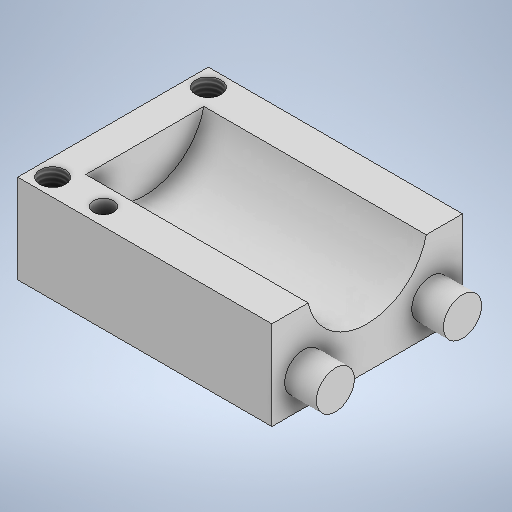
# Autodesk Inventor part: Rb oven housing bottom-back threaded
Saved by Autodesk Inventor 2025.3 (Build 293356000, 356)
## iProperties
Created: 2025-04-11
Part Number: Rb oven housing bottom-back threaded
Material: Generic
Document SubType Name: Modeling
Designer: Verðandi
Density: 1 g/cm^3
Appearance: Default
Author: Verðandi
Autodesk Inventor part; units mm, degrees
ref_plane "YZ Plane" through (0, 0, 0) normal (1, 0, 0) x (0, 1, 0)
ref_plane "XZ Plane" through (0, 0, 0) normal (0, 1, 0) x (-1, 0, 0)
ref_plane "XY Plane" through (0, 0, 0) normal (0, 0, 1) x (1, 0, 0)
sketch "Sketch1" plane through (0, 0, 0) normal (0, 0, 1) x (1, 0, 0)
  line L0 (20, -7) -> (-20, -7)
  line L1 (-20, -7) -> (-20, 7)
  line L2 (-20, 7) -> (20, 7)
  line L3 (20, 7) -> (20, -7)
  line L4 (20, -7) -> (-20, 7) construction
  line L5 (-20, -7) -> (20, 7) construction
  point P0 (0, 0)
  dimension "d0" = 40
  dimension "d1" = 14
  constraints: 12 end point, 2 midpoint, 2 parallel, 1 horizontal, 1 perpendicular
  measures "d0" distance of L1.end L2.end
  measures "d1" distance of L0.end L1.end
extrude "Extrusion1" add sketch "Sketch1" along normal blind 30
sketch "Sketch2" plane through (20, -7, 0) normal (1, 0, 0) x (0, 0, -1)
  line L0 (0, 14) -> (-30, 14) projected
  line L1 (-15, 14) -> (-15, 16)
  arc A0 (-24.2871, 14) -> (-5.7129, 14) centre (-15, 16) ccw
  point P0 (0, 7)
  dimension "d4" = 2
  dimension "d5" = 19
  constraints: 2 end point, 2 point on circle, 2 point on line, 1 centre point, 1 coincident, 1 midpoint, 1 vertical
  measures "d4" distance of L1.start L1.end
  measures "d5" diameter of A0
extrude "Extrusion2" cut sketch "Sketch2" against normal blind 35
sketch "Sketch3" plane through (-20, 7, 0) normal (0, 1, 0) x (1, 0, 0)
  line L0 (0, 0) -> (0, -30) projected
  line L1 (0, 0) -> (0, -2.75)
  line L2 (0, -2.75) -> (2.75, -2.75)
  circle A0 centre (2.75, -2.75) radius 2
  line L3 (0, -30) -> (0, -27.25)
  line L4 (0, -27.25) -> (2.75, -27.25)
  circle A1 centre (2.75, -27.25) radius 2
  point P0 (20, 0)
  dimension "d8" = 2.75
  dimension "d9" = 2.75
  dimension "d10" = 4
  dimension "d11" = 2.75
  dimension "d12" = 2.75
  dimension "d13" = 4
  constraints: 8 end point, 2 centre point, 2 coincident, 2 perpendicular, 2 point on line
  measures "d8" distance of L0.start L1.end
  measures "d9" distance of L1.end L2.end
  measures "d10" diameter of A0
  measures "d11" distance of L0.end L3.end
  measures "d12" distance of L3.end L4.end
  measures "d13" diameter of A1
extrude "Extrusion3" cut sketch "Sketch3" against normal blind 12
thread "Thread1" size "M4x0.7" class "6H" standard "ANSI Metric M Profile" full length
thread "Thread2" size "M4x0.7" class "6H" standard "ANSI Metric M Profile" full length
sketch "Sketch4" plane through (-20, 7, 0) normal (0, 1, 0) x (1, 0, 0)
  circle A0 centre (2.75, -27.25) radius 2 projected
  line L0 (2.75, -27.25) -> (10.75, -27.25)
  circle A1 centre (10.75, -27.25) radius 1.5875
  point P0 (20, 0)
  dimension "d20" = 8
  dimension "d21" = 3.175
  constraints: 2 end point, 1 centre point, 1 coincident, 1 horizontal
  measures "d20" distance of L0.start L0.end
  measures "d21" diameter of A1
extrude "Extrusion4" cut sketch "Sketch4" against normal blind 10.5 contours A1
sketch "Sketch5" plane through (20, -7, 0) normal (1, 0, 0) x (0, 0, -1)
  line L0 (0, 0) -> (-30, 0) projected
  line L1 (-30, 0) -> (-25, 0)
  line L2 (-25, 0) -> (-25, 5)
  circle A0 centre (-25, 5) radius 3
  line L3 (0, 0) -> (0, 14) projected
  line L4 (0, 0) -> (-5, 0)
  line L5 (-5, 0) -> (-5, 5)
  circle A1 centre (-5, 5) radius 3
  point P0 (0, 7)
  dimension "d24" = 5
  dimension "d25" = 5
  dimension "d26" = 6
  dimension "d27" = 5
  dimension "d28" = 5
  dimension "d29" = 6
  constraints: 8 end point, 2 centre point, 2 coincident, 2 perpendicular, 2 point on line
  measures "d24" distance of L0.end L1.end
  measures "d25" distance of L1.end L2.end
  measures "d26" diameter of A0
  measures "d27" distance of L0.start L4.end
  measures "d28" distance of L4.end L5.end
  measures "d29" diameter of A1
extrude "Extrusion5" add sketch "Sketch5" along normal blind 5
body "Solid1"
